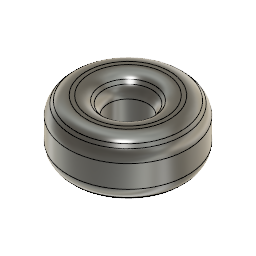
TreeStrapBead (Autodesk Fusion 360 design; units mm, degrees)
Autodesk Fusion 360 part; units mm, degrees
sketch "Sketch1" plane through (0, 0, 0) normal (0, 0, 1) x (1, 0, 0)
  circle A0 centre (0, 0) radius 1.75
  circle A1 centre (0, 0) radius 5.25
  dimension "d1" = 3.5
  dimension "d2" = 3.5
  constraint coincident A0.centre A1.centre
  measures "d1" diameter of A0
  measures "d2" distance of A0
extrude "Extrude1" add sketch "Sketch1" along normal blind 5
chamfer "Chamfer1" distance 1 angle 45 4 edges at (-1.6316, 0.6328, 5) (-4.8947, -1.8985, 5) (-4.8947, -1.8985, 0) (-1.6316, 0.6328, 0)
fillet "Fillet1" radius 1.25 4 edges at (-4.8947, -1.8985, 4) (-4.8947, 1.8985, 1) (-1.6316, 0.6328, 4) (-1.6316, -0.6328, 1)
fillet "Fillet2" radius 1.4 4 edges at (-3.9624, -1.5369, 0) (-2.5639, 0.9944, 0) (-2.5639, -0.9944, 5) (-3.9624, 1.5369, 5)
